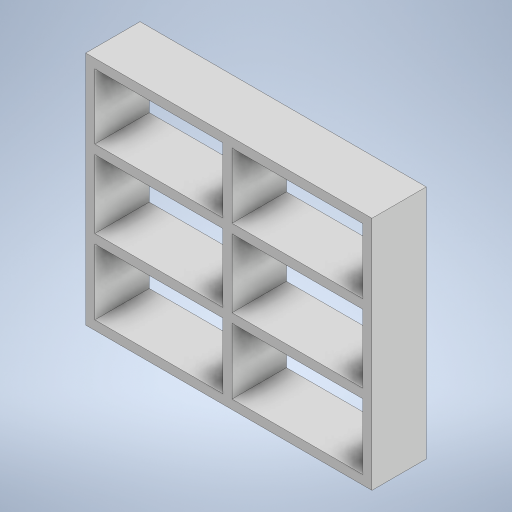
# Autodesk Inventor part: Repisa
Saved by Autodesk Inventor 2023 (Build 270158000, 158)
## iProperties
Created: 2023-06-01
Part Number: Repisa
Material: Generic
Document SubType Name: Modeling
Designer: Zenbook
Density: 1 g/cm^3
Appearance: Default
Author: Zenbook
Autodesk Inventor part; units mm, degrees
ref_plane "YZ Plane" through (0, 0, 0) normal (1, 0, 0) x (0, 1, 0)
ref_plane "XZ Plane" through (0, 0, 0) normal (0, 1, 0) x (-1, 0, 0)
ref_plane "XY Plane" through (0, 0, 0) normal (0, 0, 1) x (1, 0, 0)
sketch "Sketch1" plane through (0, 0, 0) normal (0, 0, 1) x (1, 0, 0)
  line L0 (0, 0) -> (532, 0)
  line L1 (532, 0) -> (532, 438)
  line L2 (532, 438) -> (0, 438)
  line L3 (0, 438) -> (0, 0)
  line L4 (0, 0) -> (17, 0)
  line L5 (0, 17) -> (0, 0)
  line L6 (532, 438) -> (515, 438)
  line L7 (532, 421) -> (532, 438)
  line L8 (0, 438) -> (272, 438)
  line L9 (272, 421) -> (272, 300)
  line L10 (255, 283) -> (17, 283)
  line L11 (0, 283) -> (0, 438)
  line L12 (17, 283) -> (255, 283)
  line L13 (255, 300) -> (17, 300)
  line L14 (0, 300) -> (0, 283)
  line L15 (272, 438) -> (255, 438)
  line L16 (0, 0) -> (272, 0)
  line L17 (272, 17) -> (272, 139)
  line L18 (255, 156) -> (17, 156)
  line L19 (0, 156) -> (0, 0)
  line L20 (0, 139) -> (0, 156)
  line L21 (272, 300) -> (515, 300)
  line L22 (515, 283) -> (272, 283)
  line L23 (515, 421) -> (272, 421)
  line L24 (255, 421) -> (17, 421)
  line L25 (17, 421) -> (17, 300)
  line L26 (255, 421) -> (255, 300)
  line L27 (255, 283) -> (255, 156)
  line L28 (255, 139) -> (255, 17)
  line L29 (17, 283) -> (17, 156)
  line L30 (17, 139) -> (17, 17)
  line L31 (272, 300) -> (272, 421)
  line L32 (272, 17) -> (272, 139)
  line L33 (272, 156) -> (272, 283)
  line L34 (17, 156) -> (255, 156)
  line L35 (272, 156) -> (515, 156)
  line L36 (515, 139) -> (272, 139)
  line L37 (255, 139) -> (17, 139)
  line L38 (17, 17) -> (255, 17)
  line L39 (272, 17) -> (515, 17)
  line L40 (515, 300) -> (515, 421)
  line L41 (515, 17) -> (515, 139)
  line L42 (515, 156) -> (515, 283)
  point P0 (272, 78)
  point P1 (255, 78)
  point P2 (136, 139)
  point P3 (136, 156)
  dimension "Ancho" = 532
  dimension "Alto" = 438
  dimension "Grosor" = 17
  dimension "d14" = 17
  dimension "d15" = 17
  dimension "d16" = 122
  dimension "d17" = 238
  dimension "d18" = 243
  dimension "d19" = 17
  dimension "d20" = 122
  dimension "d21" = 17
  dimension "d22" = 127
  dimension "d23" = 17
  dimension "d24" = 17
  dimension "d25" = 127
  dimension "d26" = 121
  dimension "d27" = 17
  dimension "d28" = 17
  dimension "d29" = 17
  dimension "d30" = 238
  dimension "d31" = 243
  dimension "d32" = 17
  dimension "d33" = 121
  dimension "d34" = 17
  dimension "d35" = 238
  dimension "d36" = 243
  dimension "d37" = 17
  constraints: 86 end point, 34 parallel, 12 horizontal, 12 perpendicular, 4 midpoint
  measures "Ancho" distance of L2.end L1.end
  measures "Alto" distance of L1.end L0.end
  measures "Grosor" horizontal distance of L0.start L30.end
  measures "d14" distance from line of L0 L39.end
  measures "d15" distance of point (272, 78) point (255, 78)
  measures "d16" distance of L30.start L30.end
  measures "d17" distance of L30.end L28.end
  measures "d18" distance of L17.start L39.end
  measures "d19" distance of L5.start L30.end
  measures "d20" distance of L39.end L36.start
  measures "d21" distance of point (136, 139) point (136, 156)
  measures "d22" distance of L10.end L18.end
  measures "d23" distance of L13.end L10.end
  measures "d24" distance of L36.start L35.end
  measures "d25" distance of L35.end L22.start
  measures "d26" distance of L21.end L23.start
  measures "d27" distance of L22.start L21.end
  measures "d28" horizontal distance of L0.end L39.end
  measures "d29" distance of L33.start L18.start
  measures "d30" distance of L18.start L18.end
  measures "d31" distance of L33.start L35.end
  measures "d32" distance from line of L1 L35.end
  measures "d33" distance of L24.end L13.end
  measures "d34" distance between parallel lines of L24 L2
  measures "d35" distance of L24.start L24.end
  measures "d36" distance of L23.start L9.start
  measures "d37" distance of L9.start L24.start
extrude "Extrusion1" add sketch "Sketch1" against normal blind 101
equation "\"d14\" = Grosor"
equation "\"d15\" = Grosor"
equation "\"d19\" = Grosor"
equation "\"d21\" = Grosor"
equation "\"d23\" = Grosor"
equation "\"d24\" = Grosor"
equation "\"d27\" = Grosor"
equation "\"d28\" = Grosor"
equation "\"d29\" = Grosor"
equation "\"d32\" = Grosor"
equation "\"d34\" = Grosor"
equation "\"d37\" = Grosor"
body "Solid1"
